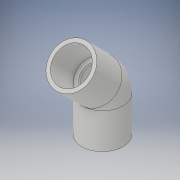
# Autodesk Inventor part: 45 Elbow 1 Inch
Saved by Autodesk Inventor 2018 (Build 220112000, 112)
## iProperties
Created: 2018-01-16
Part Number: 45 Elbow 1 Inch
Material: Generic
Document SubType Name: Modeling
Designer: owner
Density: 1 g/cm^3
Appearance: Default
Author: owner
Autodesk Inventor part; units mm, degrees
ref_plane "YZ Plane" through (0, 0, 0) normal (1, 0, 0) x (0, 1, 0)
ref_plane "XZ Plane" through (0, 0, 0) normal (0, 1, 0) x (-1, 0, 0)
ref_plane "XY Plane" through (0, 0, 0) normal (0, 0, 1) x (1, 0, 0)
sketch "Sketch1" plane through (0, 0, 0) normal (0, 1, 0) x (-1, 0, 0)
  circle A0 centre (0, 0) radius 20.3835
  dimension "d0" = 40.767
  constraints: 1 centre point, 1 coincident
  measures "d0" diameter of A0
extrude "Extrusion1" add sketch "Sketch1" along normal blind 34.7218
sketch "Sketch2" plane through (0, 34.7218, 0) normal (0, 1, 0) x (1, 0, 0)
  circle A0 centre (0, 0) radius 20.3835 projected
  line L0 (0, -20.3835) -> (-27.7458, -20.3835)
  constraints: 2 end point, 2 horizontal, 1 vertical alignment, 1 other
ref_plane "Work Plane1" through (0, 34.7218, 20.3835) normal (0, 0.7071068, 0.7071068) x (-1, 0, 0)
sketch "Sketch3" plane through (0, 34.7218, 20.3835) normal (0, 0.7071068, 0.7071068) x (-1, 0, 0)
  circle A0 centre (0, -20.3835) radius 20.3835 projected
  circle A1 centre (0, -20.3835) radius 20.3835
  point P0 (0, 10.1387)
  constraints: 1 centre point, 1 coincident
extrude "Extrusion2" add sketch "Sketch3" along normal blind 34.7218
sketch "Sketch4" plane through (0, 0, 0) normal (0, -1, 0) x (1, 0, 0)
  circle A0 centre (0, 0) radius 16.7767
  dimension "d6" = 33.5534
  constraints: 1 centre point, 1 coincident
  measures "d6" diameter of A0
extrude "Extrusion3" cut sketch "Sketch4" against normal blind 31.75
sketch "Sketch5" plane through (0, 73.6871, 30.5222) normal (0, 0.7071068, 0.7071068) x (1, 0, 0)
  circle A0 centre (0, 0) radius 16.7767
  point P0 (0, -30.5222)
  dimension "d9" = 33.5534
  constraints: 1 centre point
  measures "d9" diameter of A0
extrude "Extrusion4" cut sketch "Sketch5" against normal blind 31.75
ref_plane "Work Plane2" through (0, 51.2365, 8.0716) normal (0, 0.7071068, 0.7071068) x (1, 0, 0)
ref_plane "Work Plane3" through (0, 31.75, 0) normal (0, -1, 0) x (1, 0, 0)
revolve "Revolution1" add sketch "Sketch2" angle 45 about axis through (0, 34.7218, 20.3835) along (1, 0, 0)
ref_plane "Work Plane4" through (0, 34.7218, 20.3835) normal (-1, 0, 0) x (0, -1, 0)
sketch "Sketch6" plane through (0, 34.7218, 20.3835) normal (-1, 0, 0) x (0, -1, 0)
  line L0 (0, 33.7996) -> (-51.2396, 33.7996)
  point P0 (34.7218, -20.3835)
  constraints: 2 end point, 1 horizontal
ref_plane "Work Plane5" through (0, 34.7218, 54.1831) normal (-0.7071068, 0, -0.7071068) x (0, 1, 0)
sketch "Sketch8" plane through (0, 34.7218, 20.3835) normal (-1, 0, 0) x (0, -1, 0)
  line L0 (-28.3776, -24.1748) -> (-4.6518, -0.449) projected
  line L1 (2.9718, -3.6068) -> (2.9718, -37.1602) projected
  line L2 (-4.6518, -0.449) -> (2.9718, -3.6068)
  point P0 (34.7218, -20.3835)
  constraints: 2 end point
sketch "Sketch9" plane through (0, 31.75, 0) normal (0, -1, 0) x (1, 0, 0)
  circle A0 centre (0, 0) radius 12.7
  dimension "d17" = 25.4
  constraints: 1 centre point, 1 coincident
  measures "d17" diameter of A0
extrude "Extrusion5" cut sketch "Sketch9" against normal blind 2.9718
sketch "Sketch10" plane through (0, 51.2365, 8.0716) normal (0, 0.7071068, 0.7071068) x (1, 0, 0)
  circle A0 centre (0, 0) radius 12.7
  point P0 (0, -30.5222)
  dimension "d20" = 25.4
  constraints: 1 centre point
  measures "d20" diameter of A0
extrude "Extrusion6" cut sketch "Sketch10" against normal blind 2.9718
sketch "Sketch11" plane through (0, 34.7218, 0) normal (0, -1, 0) x (1, 0, 0)
  circle A0 centre (0, 0) radius 12.7
  line L0 (28.5369, 20.3835) -> (-28.5369, 20.3835) projected
  constraints: 1 centre point, 1 coincident
revolve "Revolution2" cut sketch "Sketch11" angle 45 about axis through (0, 34.7218, 20.3835) along (1, 0, 0)
body "Solid1"
